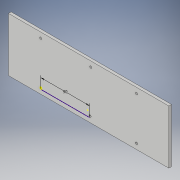
# Autodesk Inventor part: acrilesheet_base
Saved by Autodesk Inventor 2019 (Build 230136000, 136)
## iProperties
Created: 2020-03-12
Part Number: acrilesheet_base
Material: Generic
Document SubType Name: Modeling
Designer: Prajwal
Density: 1 g/cm^3
Appearance: Default
Author: Prajwal
d50: 90.000 mm
Autodesk Inventor part; units mm, degrees
ref_plane "YZ Plane" through (0, 0, 0) normal (1, 0, 0) x (0, 1, 0)
ref_plane "XZ Plane" through (0, 0, 0) normal (0, 1, 0) x (-1, 0, 0)
ref_plane "XY Plane" through (0, 0, 0) normal (0, 0, 1) x (1, 0, 0)
sketch "Sketch1" plane through (0, 0, 0) normal (0, 0, 1) x (1, 0, 0)
  line L0 (-147.4604, 81.9415) -> (150.5396, 81.9415)
  line L1 (150.5396, 81.9415) -> (150.5396, -18.0585)
  line L2 (150.5396, -18.0585) -> (-147.4604, -18.0585)
  line L3 (-147.4604, -18.0585) -> (-147.4604, 81.9415)
  point P0 (0, 0)
  constraints: 8 end point, 2 parallel, 1 horizontal, 1 perpendicular
extrude "Extrusion1" add sketch "Sketch1" along normal blind 5
sketch "Sketch2" plane through (0, 0, 5) normal (0, 0, 1) x (1, 0, 0)
  line L0 (150.5396, 81.9415) -> (-147.4604, 81.9415) projected
  line L1 (-147.4604, 81.9415) -> (-87.4604, 81.9415)
  line L2 (-87.4604, 81.9415) -> (-147.4604, 81.9415)
  line L3 (-147.4604, 81.9415) -> (-147.4604, 71.9415)
  line L4 (-147.4604, 81.9415) -> (-147.4604, -18.0585) projected
  line L5 (-147.4604, 71.9415) -> (-147.4604, 76.9415)
  line L6 (-87.4604, 81.9415) -> (-87.4604, 71.9415)
  line L7 (-87.4604, 71.9415) -> (-84.9499, 65.8304)
  point P0 (0, 0)
  dimension "d4" = 60
  dimension "d5" = 10
  dimension "d6" = 10
  constraints: 12 end point, 2 point on line, 1 collinear, 1 midpoint, 1 vertical
  measures "d4" distance of L0.end L1.end
  measures "d5" distance of L0.end L3.end
  measures "d6" distance of L1.end L6.end
hole "Hole1" at (-87.4604, 71.9415, 5) direction (0, 0, -1) diameter 4 depth 6 tip angle 118
sketch "Sketch3" plane through (0, 0, 5) normal (0, 0, 1) x (1, 0, 0)
  line L0 (150.5396, 81.9415) -> (150.5396, -18.0585) projected
  line L1 (150.5396, 81.9415) -> (90.5396, 81.9415)
  line L2 (-147.4604, 81.9415) -> (150.5396, 81.9415) projected
  line L3 (90.5396, 81.9415) -> (132.2292, 81.9415)
  line L4 (90.5396, 81.9415) -> (90.5396, 71.9415)
  line L5 (90.5396, 71.9415) -> (90.5396, 66.7383)
  point P0 (0, 0)
  dimension "d14" = 60
  dimension "d15" = 10
  constraints: 8 end point, 3 point on line, 1 perpendicular
  measures "d14" distance of L0.start L1.end
  measures "d15" distance of L1.end L4.end
hole "Hole2" at (90.5396, 71.9415, 5) direction (0, 0, -1) diameter 4 depth 6 tip angle 118
sketch "Sketch4" plane through (0, 0, 5) normal (0, 0, 1) x (1, 0, 0)
  line L0 (150.5396, -18.0585) -> (-147.4604, -18.0585) projected
  line L1 (-147.4604, -18.0585) -> (59852.5396, -18.0585)
  line L2 (-147.4604, -18.0585) -> (-147.4604, 81.9415) projected
  line L3 (59852.5396, -18.0585) -> (-147.4604, -18.0585)
  line L4 (-147.4604, -18.0585) -> (-87.4604, -18.0585)
  line L5 (-87.4604, -18.0585) -> (-147.4604, -18.0585)
  line L6 (-87.4604, -18.0585) -> (-87.4604, -8.0585)
  line L7 (-87.4604, -8.0585) -> (-87.4604, -4.3661)
  point P0 (0, 0)
  dimension "d23" = 60000
  dimension "d24" = 60
  dimension "d25" = 10
  constraints: 12 end point, 3 collinear, 2 point on line, 1 perpendicular
  measures "d23" distance of L0.end L1.end
  measures "d24" distance of L0.end L4.end
  measures "d25" distance of L4.end L6.end
hole "Hole3" at (-87.4604, -8.0585, 5) direction (0, 0, -1) diameter 4 depth 6 tip angle 118
sketch "Sketch5" plane through (0, 0, 5) normal (0, 0, 1) x (1, 0, 0)
  line L0 (150.5396, 81.9415) -> (150.5396, -18.0585) projected
  line L1 (150.5396, -18.0585) -> (90.5396, -18.0585)
  line L2 (150.5396, -18.0585) -> (-147.4604, -18.0585) projected
  line L3 (90.5396, -18.0585) -> (90.5396, -8.0585)
  line L4 (90.5396, -8.0585) -> (90.5396, -4.7819)
  point P0 (0, 0)
  dimension "d33" = 60
  dimension "d34" = 10
  constraints: 6 end point, 2 point on line, 1 vertical
  measures "d33" distance of L0.end L1.end
  measures "d34" distance of L1.end L3.end
hole "Hole4" at (90.5396, -8.0585, 5) direction (0, 0, -1) diameter 4 depth 6 tip angle 118
sketch "Sketch6" plane through (0, 0, 5) normal (0, 0, 1) x (1, 0, 0)
  circle A0 centre (-87.4604, 71.9415) radius 2 projected
  line L0 (-87.4604, 71.9415) -> (5.4056, 71.9415)
  line L1 (5.4056, 71.9415) -> (-84.5944, 71.9415)
  line L2 (-84.5944, 71.9415) -> (5.4056, 71.9415)
  point P0 (0, 0)
  dimension "d42" = 90
  constraints: 6 end point, 1 collinear, 1 horizontal, 1 point on line
  measures "d42" distance of L0.end L1.end
hole "Hole5" at (5.4056, 71.9415, 5) direction (0, 0, -1) diameter 4 depth 6 tip angle 118
sketch "Sketch7" plane through (0, 0, 5) normal (0, 0, 1) x (1, 0, 0)
  circle A0 centre (-87.4604, -8.0585) radius 2 projected
  line L0 (-87.4604, -10.0585) -> (2.9107, -10.0585)
  line L1 (2.9107, -10.0585) -> (-87.0893, -10.0585)
  point P0 (0, 0)
  dimension "d50" = 90
  constraints: 4 end point, 2 horizontal, 1 point on line, 1 vertical alignment, 1 other
  measures "d50" distance of L0.end L1.end
sketch "Sketch8" plane through (0, 0, 5) normal (0, 0, 1) x (1, 0, 0)
  point P0 (0, 0)
  point P1 (4.1582, -7.2768)
hole "Hole6" at (4.1582, -7.2768, 5) direction (0, 0, -1) diameter 4 depth 6 tip angle 118
body "Solid1"
